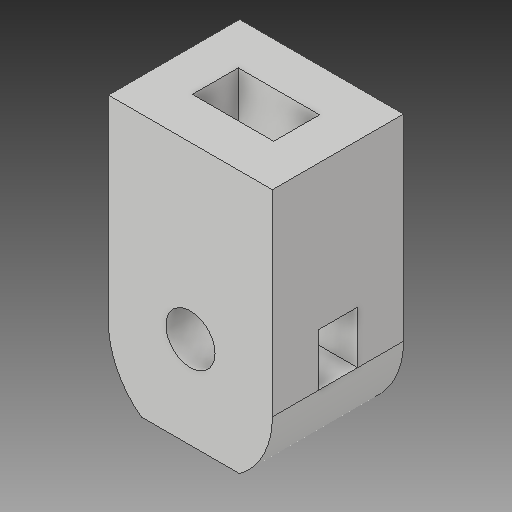
# Autodesk Inventor part: Acople tuerca salida
Saved by Autodesk Inventor 2019 (Build 230136000, 136)
## iProperties
Created: 2020-02-01
Part Number: Acople tuerca salida
Material: Generic
Document SubType Name: Modeling
Designer: Elías Sánchez
Density: 1 g/cm^3
Appearance: Default
Description: Impresión 3D
Author: Elías Sánchez
Revision Number: IR
Autodesk Inventor part; units mm, degrees
ref_plane "YZ Plane" through (0, 0, 0) normal (1, 0, 0) x (0, 1, 0)
ref_plane "XZ Plane" through (0, 0, 0) normal (0, 1, 0) x (-1, 0, 0)
sketch "Sketch1" plane through (0, 0, 0) normal (0, 0, 1) x (1, 0, 0)
  line L0 (12.5, 0) -> (12.5, 30)
  line L1 (12.5, 30) -> (-12.5, 30)
  line L2 (-12.5, 30) -> (-12.5, 0)
  arc A0 (-12.5, 0) -> (12.5, 0) centre (0, 0) ccw
  point P0 (0, 30)
  dimension "d0" = 25
  dimension "d1" = 30
  dimension "d2" = 30
  dimension "d3" = 12.5
  dimension "d4" = 12.5
  dimension "d5" = 12.5
  constraints: 6 end point, 2 coincident, 2 point on circle, 1 centre point, 1 midpoint, 1 parallel, 1 vertical alignment
  measures "d0" distance of L0.end L1.end
  measures "d1" distance of L0.start L0.end
  measures "d2" distance from line of point (0, 0) L1
  measures "d3" radius of A0
  measures "d4" distance of point (0, 0) L0.start
  measures "d5" distance from line of point (0, 0) L2
extrude "Extrusion1" add sketch "Sketch1" along normal blind 20
ref_plane "Work Plane1" through (0, 0, 10) normal (0, 0, 1) x (1, 0, 0)
sketch "Sketch2" plane through (0, 0, 10) normal (0, 0, 1) x (1, 0, 0)
  line L0 (6.2, 3.5796) -> (6.2, -3.5796)
  line L1 (6.2, -3.5796) -> (0, -7.1591)
  line L2 (0, -7.1591) -> (-6.2, -3.5796)
  line L3 (-6.2, -3.5796) -> (-6.2, 3.5796)
  line L4 (-6.2, 3.5796) -> (0, 7.1591)
  line L5 (0, 7.1591) -> (6.2, 3.5796)
  line L6 (12.5, 30) -> (12.5, 0) projected
  line L7 (-12.5, 0) -> (-12.5, 30) projected
  line L8 (-12.5, 30) -> (12.5, 30) projected
  line L9 (12.5, 30) -> (12.5, 0) projected
  arc A0 (-12.5, 0) -> (12.5, 0) centre (0, 0) ccw projected
  dimension "d9" = 12.4
  constraints: 12 end point, 1 coincident, 1 vertical, 13 other
  measures "d9" distance between parallel lines of L0 L3
extrude "Extrusion2" cut sketch "Sketch2" along normal mid plane 7 contours L0 L1 L2 L3 L4 L5
sketch "Sketch3" plane through (0, 0, 0) normal (0, 1, 0) x (-1, 0, 0)
  point P0 (0, 0)
sketch "Sketch4" plane through (0, 0, 10) normal (0, 0, 1) x (1, 0, 0)
  point P0 (0, 0)
sketch "Sketch6" plane through (0, 0, 0) normal (0, 1, 0) x (-1, 0, 0)
  line L0 (6.2, 13.5) -> (6.2, 6.5) projected
  line L1 (0, 13.5) -> (-6.2, 13.5) projected
  line L2 (6.2, 6.5) -> (-6.2, 6.5)
  line L3 (-6.2, 6.5) -> (-6.2, 13.5)
  line L4 (-6.2, 13.5) -> (6.2, 13.5)
  line L5 (6.2, 13.5) -> (6.2, 6.5)
  point P0 (0, 0)
  constraints: 8 end point, 2 parallel, 1 horizontal, 1 perpendicular
extrude "Extrusion3" cut sketch "Sketch6" along normal blind 30
sketch "Sketch7" plane through (0, 0, 20) normal (0, 0, 1) x (1, 0, 0)
  arc A0 (-12.5, 0) -> (12.5, 0) centre (0, 0) ccw projected
  line L0 (12.5, 30) -> (-12.5, 30) projected
  line L1 (12.5, 0) -> (12.5, 30) projected
  point P0 (0, 4)
  dimension "d27" = 26
  dimension "d28" = 12.5
  constraints: 1 coincident
  measures "d27" distance from line of L0 point (0, 4)
  measures "d28" distance from line of L1 point (0, 4)
hole "Hole1" at (0, 4, 20) direction (0, 0, -1) diameter 7.5 end through all
sketch "Sketch8" plane through (-12.5, 0, 0) normal (-1, 0, 0) x (0, 0, 1)
  line L0 (7, 8) -> (13, 8)
  line L1 (13, 8) -> (13, 0)
  line L2 (13, 0) -> (7, 0)
  line L3 (7, 0) -> (7, 8)
  line L4 (0, 0) -> (0, 30) projected
  dimension "d21" = 6
  dimension "d22" = 8
  dimension "d23" = 7
  dimension "d24" = 0
  constraints: 8 end point, 2 parallel, 1 horizontal, 1 perpendicular
  measures "d21" distance between parallel lines of L1 L3
  measures "d22" distance between parallel lines of L2 L0
  measures "d23" distance between parallel lines of L4 L3
  measures "d24" distance from line of L4.start L2
extrude "Extrusion4" cut sketch "Sketch8" against normal blind 25
sketch "Sketch9" plane through (0, 0, 20) normal (0, 0, 1) x (1, 0, 0)
  line L0 (-10, -10) -> (10, -10)
  line L1 (10, -10) -> (10, -15)
  line L2 (10, -15) -> (-10, -15)
  line L3 (-10, -15) -> (-10, -10)
  point P0 (0, 0)
  point P1 (0, -10)
  dimension "d29" = 10
  dimension "d30" = 5
  dimension "d31" = 20
  constraints: 8 end point, 2 parallel, 1 horizontal, 1 midpoint, 1 perpendicular, 1 vertical alignment
  measures "d29" distance from line of point (0, 0) L0
  measures "d30" distance between parallel lines of L0 L2
  measures "d31" distance between parallel lines of L1 L3
extrude "Extrusion5" cut sketch "Sketch9" against normal blind 20
equation "\"d1\" = d2"
body "Solid1"
